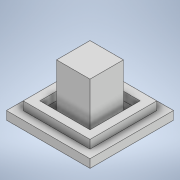
# Autodesk Inventor part: latticeChamberCapv4
Saved by Autodesk Inventor 2020.5 (Build 245400000, 400)
## iProperties
Created: 2022-09-15
Part Number: latticeChamberCapv4
Material: Generic
Document SubType Name: Modeling
Designer: kouda
Density: 1 g/cm^3
Appearance: Default
Author: kouda
Autodesk Inventor part; units mm, degrees
ref_plane "YZ Plane" through (0, 0, 0) normal (1, 0, 0) x (0, 1, 0)
ref_plane "XZ Plane" through (0, 0, 0) normal (0, 1, 0) x (-1, 0, 0)
ref_plane "XY Plane" through (0, 0, 0) normal (0, 0, 1) x (1, 0, 0)
sketch "Sketch1" plane through (0, 0, 0) normal (0, 1, 0) x (-1, 0, 0)
  line L0 (0, 0) -> (20, 0)
  line L1 (20, 0) -> (20, -20)
  line L2 (20, -20) -> (0, -20)
  line L3 (0, -20) -> (0, 0)
  dimension "d0" = 20
  dimension "d1" = 20
  constraints: 8 end point, 2 parallel, 1 horizontal, 1 perpendicular
  measures "d0" distance of L1.end L2.end
  measures "d1" distance of L0.end L1.end
extrude "Extrusion1" add sketch "Sketch1" along normal blind 2
sketch "Sketch2" plane through (0, 2, 0) normal (0, 1, 0) x (1, 0, 0)
  line L0 (0, 20) -> (-20, 20) projected
  line L1 (-20, 20) -> (-20, 0) projected
  line L2 (-20, 0) -> (0, 0) projected
  line L3 (0, 0) -> (0, 20) projected
  line L4 (-18, 2) -> (-18, 18)
  line L5 (-18, 18) -> (-2, 18)
  line L6 (-2, 18) -> (-2, 2)
  line L7 (-2, 2) -> (-18, 2)
  line L8 (-16, 16) -> (-16, 4)
  line L9 (-16, 4) -> (-4, 4)
  line L10 (-4, 4) -> (-4, 16)
  line L11 (-4, 16) -> (-16, 16)
  dimension "d4" = 2
  dimension "d5" = 2
  constraints: 16 end point, 6 other
  measures "d4" distance between parallel lines of L1 L4
  measures "d5" distance between parallel lines of L4 L8
extrude "Extrusion2" add sketch "Sketch2" along normal blind 2 contours L4 L5 L6 L7
extrude "Extrusion3" cut sketch "Sketch2" against normal blind 10 contours L11 L10 L9 L8
sketch "Sketch3" plane through (0, 0, 0) normal (0, -1, 0) x (1, 0, 0)
  line L0 (-4, -4) -> (-4, -16) projected
  line L1 (-4, -16) -> (-16, -16) projected
  line L2 (-16, -16) -> (-16, -4) projected
  line L3 (-16, -4) -> (-4, -4) projected
  line L4 (0, -20) -> (-20, -20) projected
  line L5 (0, 0) -> (0, -20) projected
  line L6 (-20, 0) -> (0, 0) projected
  line L7 (-20, -20) -> (-20, 0) projected
  line L8 (-6, -6) -> (-6, -14)
  line L9 (-6, -14) -> (-14, -14)
  line L10 (-14, -14) -> (-14, -6)
  line L11 (-14, -6) -> (-6, -6)
  constraints: 8 end point, 3 other
extrude "Extrusion4" add sketch "Sketch3" against normal up to surface (2 mm away) contours L0 L1 L2 L3
extrude "Extrusion5" add sketch "Sketch3" against normal blind 12.5 contours L8 L9 L10 L11
body "Solid1"
